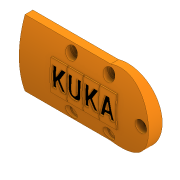
# Autodesk Inventor part: 5th Axis Cover
Saved by Autodesk Inventor 2020 (Build 240168000, 168)
## iProperties
Created: 2021-06-30
Part Number: 5th Axis Cover
Material: Generic
Document SubType Name: Modeling
Designer: Coy
Density: 1 g/cm^3
Appearance: Orange
Author: Coy
Autodesk Inventor part; units mm, degrees
ref_plane "YZ Plane" through (0, 0, 0) normal (1, 0, 0) x (0, 1, 0)
ref_plane "XZ Plane" through (0, 0, 0) normal (0, 1, 0) x (-1, 0, 0)
ref_plane "XY Plane" through (0, 0, 0) normal (0, 0, 1) x (1, 0, 0)
sketch "Sketch1" plane through (0, 0, 0) normal (0, 0, 1) x (1, 0, 0)
  arc A0 (38.3751, 46.0296) -> (50.3749, 46.0296) centre (44.375, 46) ccw
  line L0 (52.0319, 48) -> (50.3749, 46.0296)
  line L1 (52.0319, 48) -> (66.1349, 48)
  line L2 (67.7919, 46.0296) -> (66.1349, 48)
  arc A1 (67.7919, 46.0296) -> (79.6954, 47.0712) centre (73.7918, 46) ccw
  line L3 (81.0149, 48.9942) -> (79.6954, 47.0712)
  arc A2 (102.144, 33.7806) -> (81.0149, 48.9942) centre (80.5, 26) ccw
  line L4 (100.7397, 31.9516) -> (102.144, 33.7806)
  arc A3 (100.7397, 31.9516) -> (100.7397, 20.0484) centre (101.5, 26) ccw
  line L5 (102.144, 18.2194) -> (100.7397, 20.0484)
  arc A4 (81.0149, 3.0058) -> (102.144, 18.2194) centre (80.5, 26) ccw
  line L6 (79.6954, 4.9288) -> (81.0149, 3.0058)
  arc A5 (79.6954, 4.9288) -> (67.7919, 5.9704) centre (73.7918, 6) ccw
  line L7 (66.1349, 4) -> (67.7919, 5.9704)
  line L8 (66.1349, 4) -> (52.0319, 4)
  line L9 (50.3749, 5.9704) -> (52.0319, 4)
  arc A6 (50.3749, 5.9704) -> (38.3751, 5.9704) centre (44.375, 6) ccw
  line L10 (36.7181, 4) -> (38.3751, 5.9704)
  line L11 (36.7181, 4) -> (10, 4)
  line L12 (6, 0) -> (6, 4)
  line L13 (6, 0) -> (73.2199, 0)
  arc A7 (73.2199, 0) -> (73.2199, 52) centre (80.5, 26) ccw
  line L14 (73.2199, 52) -> (6, 52)
  line L15 (6, 48) -> (6, 52)
  line L16 (10, 48) -> (36.7181, 48)
  line L17 (38.3751, 46.0296) -> (36.7181, 48)
  line L18 (6, 48) -> (6, 4)
  line L19 (10, 48) -> (10, 4)
  circle A8 centre (44.375, 46) radius 3
  circle A9 centre (73.7918, 46) radius 3
  circle A10 centre (44.375, 6) radius 3
  circle A11 centre (73.7918, 6) radius 3
  circle A12 centre (101.5, 26) radius 3
  point P0 (0, 0)
  point P1 (-24, 26)
  dimension "d0" = 4
  dimension "d1" = 6
  dimension "d2" = 6
  dimension "d3" = 6
  dimension "d4" = 6
  dimension "d5" = 6
  constraints: 40 end point, 16 point on circle, 13 centre point, 3 coincident, 1 parallel, 1 vertical
  measures "d0" distance between parallel lines of L18 L19
  measures "d1" diameter of A8
  measures "d2" diameter of A9
  measures "d3" diameter of A10
  measures "d4" diameter of A11
  measures "d5" diameter of A12
extrude "Extrusion1" add sketch "Sketch1" along normal blind 5.75
sketch "Sketch2" plane through (0, 0, 5.75) normal (0, 0, 1) x (1, 0, 0)
  line L0 (73.2199, 52) -> (6, 52) projected
  line L1 (6, 52) -> (6, 0) projected
  line L2 (6, 0) -> (73.2199, 0) projected
  arc A0 (73.2199, 0) -> (73.2199, 52) centre (80.5, 26) ccw projected
  circle A1 centre (73.7918, 46) radius 3 projected
  circle A2 centre (44.375, 46) radius 3 projected
  circle A3 centre (101.5, 26) radius 3 projected
  circle A4 centre (73.7918, 6) radius 3 projected
  circle A5 centre (44.375, 6) radius 3 projected
  point P0 (0, 0)
extrude "Extrusion2" add sketch "Sketch2" along normal blind 5
sketch "Sketch3" plane through (6, 0, 0) normal (-1, 0, 0) x (0, 0, 1)
  line L0 (5.75, 67.7899) -> (5.75, -18.476) construction
  line L1 (10.75, 52) -> (10.75, 0) construction
  line L2 (0, -1) -> (10.75, -1) construction
  line L3 (0, 53) -> (10.75, 53) projected
  line L4 (10.75, -1) -> (10.75, 53) projected
  line L5 (0, -1) -> (10.75, -1) projected
  line L6 (0, -1) -> (10.75, -1) projected
  line L7 (0, 53) -> (10.75, 53) projected
  arc A0 (5.75, -1) -> (5.75, 53) centre (-64.65, 26) ccw
  line L8 (10.75, 29) -> (10.75, 23) projected
  point P0 (0, 0)
  point P1 (10.75, 26)
  point P2 (5.75, -1)
  point P3 (5.75, 53)
  dimension "d10" = 5
  constraints: 4 point on line, 2 end point, 2 point on circle, 1 centre point, 1 tangent, 1 vertical
  measures "d10" distance between parallel lines of L1 L0
extrude "Extrusion3" cut sketch "Sketch3" against normal through all
fillet "Fillet1" radius 2 7 edges at (93.9394, 44.665, 5.75) (93.9394, 7.335, 5.75) (59.0834, 48, 5.75) (59.0834, 4, 5.75) (23.3591, 4, 5.75) (23.3591, 48, 5.75) (10, 26, 5.75)
ref_plane "Work Plane1" through (6, 26, 10.75) normal (0, 0, -1) x (-1, 0, 0)
sketch "Sketch4" plane through (6, 26, 10.75) normal (0, 0, -1) x (-1, 0, 0)
  line L0 (0, -26) -> (0, 26) construction
  line L1 (-67.2199, -26) -> (0, -26) construction
  line L2 (0, 26) -> (-67.2199, 26) construction
  line L3 (-25, 12) -> (-76.5, 12)
  line L4 (-76.5, 12) -> (-76.5, -12)
  line L5 (-76.5, -12) -> (-25, -12)
  line L6 (-25, -12) -> (-25, 12)
  point P0 (6, -26)
  dimension "d14" = 14
  dimension "d15" = 14
  dimension "d16" = 25
  dimension "d17" = 25
  constraints: 8 end point, 2 horizontal alignment, 2 parallel, 1 horizontal, 1 perpendicular, 8 other
  measures "d14" distance between parallel lines of L2 L3
  measures "d15" distance between parallel lines of L1 L5
  measures "d16" distance from line of point (-101.5, 0) L4
  measures "d17" distance between parallel lines of L0 L6
extrude "Extrusion4" add sketch "Sketch4" along normal mid plane 2
sketch "Sketch5" plane through (6, 26, 11.75) normal (0, 0, 1) x (1, 0, 0)
  line L0 (25.0625, 11.9604) -> (75.7338, 11.9604) construction
  line L1 (75.7338, 11.9604) -> (75.7338, -11.8038) construction
  line L2 (75.7338, -11.8038) -> (25.0625, -11.8038) construction
  line L3 (25.0625, -11.8038) -> (25.0625, 11.9604) construction
  line L4 (37.2371, -7.3812) -> (33.5938, -7.3812)
  line L5 (33.5938, -7.3812) -> (30.3211, -1.1814)
  line L6 (30.3211, -1.1814) -> (29.7283, -2.2312)
  line L7 (29.7283, -2.2312) -> (29.7283, -7.3812)
  line L8 (29.7283, -7.3812) -> (26.7025, -7.3812)
  line L9 (26.7025, -7.3812) -> (26.7025, 7.8588)
  line L10 (26.7025, 7.8588) -> (29.7283, 7.8588)
  line L11 (29.7283, 7.8588) -> (29.7283, 1.0663)
  line L12 (29.7283, 1.0663) -> (33.5815, 7.8588)
  line L13 (33.5815, 7.8588) -> (37.0642, 7.8588)
  line L14 (37.0642, 7.8588) -> (32.7787, 0.7822)
  line L15 (32.7787, 0.7822) -> (37.2371, -7.3812)
  spline S0 degree 2 poles (43.8732, -7.7023) (41.4526, -7.7023) (38.8467, -4.7383) (38.8467, -1.873) knots 0 0 0 1 2 2 2
  line L16 (38.8467, -1.873) -> (38.8467, 7.8588)
  line L17 (38.8467, 7.8588) -> (41.8725, 7.8588)
  line L18 (41.8725, 7.8588) -> (41.8725, -1.6507)
  spline S1 degree 2 poles (41.8725, -1.6507) (41.8725, -3.2439) (42.8111, -4.8) (43.8732, -4.8) knots 0 0 0 1 2 2 2
  spline S2 degree 2 poles (43.8732, -4.8) (44.9106, -4.8) (45.8863, -3.3056) (45.8863, -1.6507) knots 0 0 0 1 2 2 2
  line L19 (45.8863, -1.6507) -> (45.8863, 7.8588)
  line L20 (45.8863, 7.8588) -> (48.912, 7.8588)
  line L21 (48.912, 7.8588) -> (48.912, -1.8607)
  spline S3 degree 2 poles (48.912, -1.8607) (48.912, -4.6765) (46.3679, -7.7023) (43.8732, -7.7023) knots 0 0 0 1 2 2 2
  line L22 (62.5753, -7.3812) -> (58.9321, -7.3812)
  line L23 (58.9321, -7.3812) -> (55.6593, -1.1814)
  line L24 (55.6593, -1.1814) -> (55.0665, -2.2312)
  line L25 (55.0665, -2.2312) -> (55.0665, -7.3812)
  line L26 (55.0665, -7.3812) -> (52.0407, -7.3812)
  line L27 (52.0407, -7.3812) -> (52.0407, 7.8588)
  line L28 (52.0407, 7.8588) -> (55.0665, 7.8588)
  line L29 (55.0665, 7.8588) -> (55.0665, 1.0663)
  line L30 (55.0665, 1.0663) -> (58.9197, 7.8588)
  line L31 (58.9197, 7.8588) -> (62.4024, 7.8588)
  line L32 (62.4024, 7.8588) -> (58.117, 0.7822)
  line L33 (58.117, 0.7822) -> (62.5753, -7.3812)
  line L34 (63.868, -7.3812) -> (67.9312, 7.8588)
  line L35 (67.9312, 7.8588) -> (71.2286, 7.8588)
  line L36 (71.2286, 7.8588) -> (75.2918, -7.3812)
  line L37 (75.2918, -7.3812) -> (72.1919, -7.3812)
  line L38 (72.1919, -7.3812) -> (71.4386, -4.269)
  line L39 (71.4386, -4.269) -> (67.6471, -4.269)
  line L40 (67.6471, -4.269) -> (66.8938, -7.3812)
  line L41 (66.8938, -7.3812) -> (63.868, -7.3812)
  line L42 (70.7717, -1.5025) -> (69.5367, 3.5363)
  line L43 (69.5367, 3.5363) -> (68.314, -1.5025)
  line L44 (68.314, -1.5025) -> (70.7717, -1.5025)
  point P0 (-6, -26)
  constraints: 2 other
sketch "Sketch6" plane through (6, 26, 11.75) normal (0, 0, 1) x (1, 0, 0)
  line L0 (25, 12) -> (76.5, 12) projected
  line L1 (37.7369, 12) -> (37.7369, -12)
  line L2 (76.5, -12) -> (25, -12) projected
  line L3 (38.2369, 12) -> (38.2369, -12)
  line L4 (50.7398, 12) -> (50.7398, -12)
  line L5 (50.2398, 12) -> (50.2398, -12.0366)
  line L6 (62.9301, 12) -> (62.9301, -12)
  line L7 (63.4301, 12) -> (63.4301, -12)
  point P0 (-6, -26)
  point P1 (63.4301, -12)
  point P2 (50.2398, -12)
  dimension "d20" = 0.5
  dimension "d21" = 0.5
  dimension "d22" = 0.5
  constraints: 12 end point, 9 point on line, 3 parallel, 2 perpendicular, 1 vertical
  measures "d20" distance between parallel lines of L1 L3
  measures "d21" distance between parallel lines of L4 L5
  measures "d22" distance between parallel lines of L6 L7
extrude "Extrusion5" cut sketch "Sketch6" against normal through all contours L0 L3 L2 L1 | L0 L4 L2 L5 | L0 L7 L2 L6
sketch "Sketch7" plane through (6, 0, 0) normal (-1, 0, 0) x (0, 0, 1)
  arc A0 (6.1254, 0) -> (6.1254, 52) centre (-64.65, 26) ccw projected
  line L0 (5.75, 46) -> (5.75, 6) projected
  line L1 (11.75, 38) -> (9.789, 38) projected
  line L2 (5.75, 38) -> (5.75, 14) projected
  line L3 (9.789, 38) -> (5.75, 38)
  line L4 (9.789, 14) -> (11.75, 14) projected
  line L5 (9.789, 14) -> (5.75, 14)
  point P0 (0, 0)
  constraints: 4 end point, 2 perpendicular
extrude "Extrusion6" add sketch "Sketch7" against normal up to surface (76.5 mm away)
sketch "Sketch8" plane through (31, 26, -64.65) normal (-1, 0, 0) x (0, 0, 1)
  arc A0 (70.7754, -26) -> (70.7754, 26) centre (0, 0) ccw projected
  arc A1 (71.7021, -26.3404) -> (71.7021, 26.3404) centre (0, 0) ccw
  line L0 (76.4, 12) -> (74.439, 12) projected
  line L1 (75.4195, 12) -> (76.4, 12)
  line L2 (74.439, -12) -> (76.4, -12) projected
  line L3 (76.4, 12) -> (76.4, -12)
  line L4 (76.4, -12) -> (75.4195, -12)
  point P0 (64.65, -26)
  point P1 (75.4387, 12)
  point P2 (75.4387, -12)
  constraints: 6 end point, 2 perpendicular, 2 point on circle, 1 centre point, 1 collinear, 1 midpoint
extrude "Extrusion7" cut sketch "Sketch8" against normal through all contours A1 L0 L3 L2
emboss "Emboss1" sketch "Sketch5" operation cut depth 1 direction (0, 0, 1) wrap yes faces at (39.4912, 32.6858, 11.444)
ref_plane "Work Plane2" through (6, 26, 10.75) normal (0, 0, -1) x (-1, 0, 0)
sketch "Sketch9" plane through (6, 26, 10.75) normal (0, 0, -1) x (-1, 0, 0)
  circle A0 centre (-38.375, 20) radius 3 projected
  circle A1 centre (-38.375, 20) radius 4.5
  circle A2 centre (-67.7918, 20) radius 3 projected
  circle A3 centre (-67.7918, 20) radius 4.5
  circle A4 centre (-67.7918, -20) radius 3 projected
  circle A5 centre (-67.7918, -20) radius 4.5
  circle A6 centre (-38.375, -20) radius 4.5
  circle A7 centre (-95.5, 0) radius 3 projected
  circle A8 centre (-95.5, 0) radius 4.5
  point P0 (6, -26)
  dimension "d31" = 9
  dimension "d32" = 9
  dimension "d33" = 9
  dimension "d34" = 9
  dimension "d35" = 9
  constraints: 5 centre point, 4 coincident, 3 vertical alignment, 2 horizontal alignment, 4 other
  measures "d31" diameter of A1
  measures "d32" diameter of A3
  measures "d33" diameter of A8
  measures "d34" diameter of A5
  measures "d35" diameter of A6
extrude "Extrusion8" cut sketch "Sketch9" against normal mid plane 12
sketch "Sketch10" plane through (0, 0, 0) normal (0, 0, 1) x (1, 0, 0)
  circle A0 centre (101.5, 26) radius 3.5
  circle A1 centre (73.7918, 46) radius 3.5
  line L0 (4, 0) -> (4, 52)
  line L1 (4, 0) -> (73.2199, 0)
  arc A2 (73.2199, 0) -> (73.2199, 52) centre (80.5, 26) ccw
  line L2 (73.2199, 52) -> (4, 52)
  circle A3 centre (73.7918, 6) radius 3.5
  circle A4 centre (44.375, 46) radius 3.5
  circle A5 centre (44.375, 6) radius 3.5
  arc A6 (38.7181, 44) -> (50.3749, 46.0296) centre (44.375, 46) ccw
  line L3 (52.0319, 48) -> (50.3749, 46.0296)
  line L4 (52.0319, 48) -> (66.1349, 48)
  line L5 (67.7919, 46.0296) -> (66.1349, 48)
  arc A7 (67.7919, 46.0296) -> (79.6954, 47.0712) centre (73.7918, 46) ccw
  line L6 (81.0149, 48.9942) -> (79.6954, 47.0712)
  arc A8 (102.144, 33.7806) -> (81.0149, 48.9942) centre (80.5, 26) ccw
  line L7 (100.7397, 31.9516) -> (102.144, 33.7806)
  arc A9 (100.7397, 31.9516) -> (100.7397, 20.0484) centre (101.5, 26) ccw
  line L8 (102.144, 18.2194) -> (100.7397, 20.0484)
  arc A10 (81.0149, 3.0058) -> (102.144, 18.2194) centre (80.5, 26) ccw
  line L9 (79.6954, 4.9288) -> (81.0149, 3.0058)
  arc A11 (79.6954, 4.9288) -> (67.7919, 5.9704) centre (73.7918, 6) ccw
  line L10 (66.1349, 4) -> (67.7919, 5.9704)
  line L11 (66.1349, 4) -> (52.0319, 4)
  line L12 (50.3749, 5.9704) -> (52.0319, 4)
  arc A12 (50.3749, 5.9704) -> (38.7181, 8) centre (44.375, 6) ccw
  line L13 (8, 8) -> (38.7181, 8)
  arc A13 (6, 10) -> (8, 8) centre (8, 10) ccw
  line L14 (6, 10) -> (6, 42)
  arc A14 (8, 44) -> (6, 42) centre (8, 42) ccw
  line L15 (38.7181, 44) -> (8, 44)
  line L16 (50.3749, 5.9704) -> (52.0319, 4)
  line L17 (66.1349, 4) -> (52.0319, 4)
  line L18 (66.1349, 4) -> (67.7919, 5.9704)
  arc A15 (79.6954, 4.9288) -> (67.7919, 5.9704) centre (73.7918, 6) ccw
  line L19 (79.6954, 4.9288) -> (81.0149, 3.0058)
  arc A16 (81.0149, 3.0058) -> (102.144, 18.2194) centre (80.5, 26) ccw
  line L20 (102.144, 18.2194) -> (100.7397, 20.0484)
  arc A17 (100.7397, 31.9516) -> (100.7397, 20.0484) centre (101.5, 26) ccw
  line L21 (100.7397, 31.9516) -> (102.144, 33.7806)
  arc A18 (102.144, 33.7806) -> (81.0149, 48.9942) centre (80.5, 26) ccw
  line L22 (81.0149, 48.9942) -> (79.6954, 47.0712)
  arc A19 (67.7919, 46.0296) -> (79.6954, 47.0712) centre (73.7918, 46) ccw
  line L23 (67.7919, 46.0296) -> (66.1349, 48)
  line L24 (66.1349, 48) -> (52.0319, 48)
  line L25 (52.0319, 48) -> (50.3749, 46.0296)
  arc A20 (38.7181, 48) -> (50.3749, 46.0296) centre (44.375, 46) ccw
  line L26 (38.7181, 48) -> (31.1328, 48)
  arc A21 (31.1328, 4) -> (31.1328, 48) centre (21.4167, 26) ccw
  line L27 (38.7181, 4) -> (31.1328, 4)
  arc A22 (50.3749, 5.9704) -> (38.7181, 4) centre (44.375, 6) ccw
  arc A23 (68.033, 32.9623) -> (68.033, 19.0377) centre (80.5, 26) ccw
  line L28 (68.033, 32.9623) -> (68.2781, 32.8254)
  arc A24 (68.2781, 32.8254) -> (68.4769, 33.1725) centre (68.3756, 33) ccw
  line L29 (68.4769, 33.1725) -> (68.237, 33.3156)
  arc A25 (80.296, 40.2779) -> (68.237, 33.3156) centre (80.5, 26) ccw
  line L30 (80.296, 40.2779) -> (80.3, 39.9986)
  arc A26 (80.3, 39.9986) -> (80.7, 39.9986) centre (80.5, 40) ccw
  line L31 (80.7, 39.9986) -> (80.704, 40.2779)
  arc A27 (92.763, 33.3156) -> (80.704, 40.2779) centre (80.5, 26) ccw
  line L32 (92.763, 33.3156) -> (92.5219, 33.1718)
  arc A28 (92.5219, 33.1718) -> (92.7231, 32.8261) centre (92.6244, 33) ccw
  line L33 (92.7231, 32.8261) -> (92.967, 32.9623)
  arc A29 (92.967, 19.0377) -> (92.967, 32.9623) centre (80.5, 26) ccw
  line L34 (92.967, 19.0377) -> (92.7219, 19.1746)
  arc A30 (92.7219, 19.1746) -> (92.5231, 18.8275) centre (92.6244, 19) ccw
  line L35 (92.5231, 18.8275) -> (92.763, 18.6844)
  arc A31 (80.704, 11.7221) -> (92.763, 18.6844) centre (80.5, 26) ccw
  line L36 (80.704, 11.7221) -> (80.7, 12.0029)
  arc A32 (80.7, 12.0029) -> (80.3, 12.0014) centre (80.5, 12) ccw
  line L37 (80.3, 12.0014) -> (80.296, 11.7221)
  arc A33 (68.237, 18.6844) -> (80.296, 11.7221) centre (80.5, 26) ccw
  line L38 (68.237, 18.6844) -> (68.4781, 18.8282)
  arc A34 (68.4781, 18.8282) -> (68.2769, 19.1739) centre (68.3756, 19) ccw
  line L39 (68.2769, 19.1739) -> (68.033, 19.0377)
  circle A35 centre (80.5, 26) radius 4
  circle A36 centre (80.5, 26) radius 7
  point P0 (0, 0)
  point P1 (-24, 26)
  dimension "d38" = 8
  dimension "d39" = 14
  constraints: 80 end point, 60 point on circle, 37 centre point, 2 coincident
  measures "d38" diameter of A35
  measures "d39" diameter of A36
extrude "Extrusion9" add sketch "Sketch10" along normal blind 2.5 contours A36
sketch "Sketch11" plane through (80.5, 26, 2.5) normal (0, 0, 1) x (1, 0, 0)
  circle A0 centre (0, 0) radius 7 projected
  point P0 (-80.5, -26)
extrude "Extrusion10" add sketch "Sketch11" along normal up to next
sketch "Sketch12" plane through (80.5, 26, 2.5) normal (0, 0, -1) x (-1, 0, 0)
  circle A0 centre (0, 0) radius 3
  point P0 (80.5, -26)
  dimension "d44" = 6
  constraints: 1 centre point
  measures "d44" diameter of A0
extrude "Extrusion11" cut sketch "Sketch12" against normal blind 1
equation "\"d15\" = d14"
equation "\"d17\" = d16"
equation "\"d32\" = d31"
equation "\"d33\" = d31"
equation "\"d34\" = d31"
equation "\"d35\" = d31"
body "Solid1"
